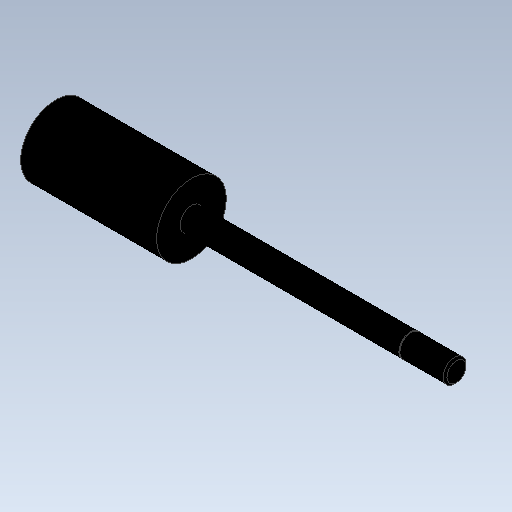
# Autodesk Inventor part: C-041.50000_rod
Saved by Autodesk Inventor 2020 (Build 240168000, 168)
## iProperties
Part Number: C-041.50000_rod
Material: Generic
Catalog Web Link: www.cadenas.de
Description: Standard Air Cylinder_rod-Original Line - Standard Air Cylinders
Vendor: BIMBA
Document SubType Name: Modeling
Designer: partserver
Manufacturer: BIMBA
Mass: 13.1943 g
Surface Area: 43.0398 cm^2
Volume: 13.1943 cm^3
Density: 1 g/cm^3
Appearance: PSOLRGB-0-0-0
Category: PARTsolutions
Company: BIMBA
PSOL_IDENT_0: {$CADENAS_DATA\23d-libs\bimba\bimba_brand\bimba_imperial\bimba_full_line\original_line_cylinders\sta
PSOL_IDENT_1: ndard_air_cylinders\rod.prj},331 {VTYP=3D},{NB=C-041.50000_rod},{LINA=C-041.50000_rod},{NN=Standard
PSOL_IDENT_2: Air Cylinder_rod},{DATE=19.01.2022 10:19:37},{GEOMDATE=27.08.2019 11:00:52},{VERSION=},{LINEID=50},{
PSOL_IDENT_3: WBVAR=STROKE,ACTING,MNT,DER,NR,BM,CO,M,EE,EEL,K,Q,Y,F,G,T,B,H,SER,SR,NT,W,E,HL,ST,STP,PRC,PB,COLOR1,
PSOL_IDENT_4: FCD,RCD,BCD,ZHJ},{WBNUMERIC=STROKE,EEL,COLOR1,FCD,RCD,BCD,ZHJ}  {NB=C-041.50000_rod},{LINA=C-041.500
PSOL_IDENT_5: 00_rod},{KT=DUMMY},{PN=C-041.5000},{DASH=},{BORE=0.75000000},{BOREPN=04},{STROKE=1.500},{STROKEALG=[
PSOL_IDENT_6: 0.001:50/0.001]},{STROKE1=1.500},{ACTING=},{ACTINGALG= '' , 'Single Acting' , 'R' , 'Reverse Single
PSOL_IDENT_7: Acting' , 'D' , 'Double Acting' },{ACTINGPN=},{MNT=},{MNTALG= '' , 'Front Nose Mounting' , 'P' , 'Re
PSOL_IDENT_8: ar Pivot Mounting' , 'BF' , 'Front Block Mounting' , 'BR' , 'Rear Block Mounting for Vertical Positi
PSOL_IDENT_9: oning' , 'BFT' , 'Front Block Trunnion Mounting' , 'BRT' , 'Rear Block Trunnion Mounting' , 'A' , 'D
PSOL_IDENT_10: ouble End Mounting with Brackets and Adjustable Stroke' , 'AP' , 'Rear Pivot Mounting with Adjustabl
PSOL_IDENT_11: e Stroke' },{TYPE=C-},{MNTPN=},{DER=},{DERALG= '' , 'N/A' },{NR=},{NRALG= '' , 'Standard' , 'NR' , '
PSOL_IDENT_12: Non-rotating - Hexagon Rod' },{NRPN=},{BM=},{BMALG= '' , 'Without Built-in Midget 3-Way Solenoid Ope
PSOL_IDENT_13: rated Valve' , 'LS' , 'With Built-in Midget 3-Way Solenoid Operated Valve' },{BMPN=},{CO=},{COALG= ''
PSOL_IDENT_14: , 'N/A' },{M=},{MALG= '', 'Without Magnet', 'M', 'With Magnet' },{EE=},{EEL=0},{EEMAX=10},{EEALG= ''
PSOL_IDENT_15: , 'Without Extra Extension', 'EE', 'With Extra Extension' },{EELALG=0},{EEPN=},{EEPN1=0.000},{K=},{K
PSOL_IDENT_16: ALG= '' , 'N/A' },{KPN=},{Q=},{QALG= '' , 'Without Side Ported Rear Head' , 'Q' , 'With Side Ported
PSOL_IDENT_17: Rear Head' },{QPN=},{Y=},{YALG= '' , 'N/A' },{YPN=},{F=},{FALG= '', 'Standard', 'F', 'Molycoated Bod
PSOL_IDENT_18: y' },{FPN=},{G=},{GPN=},{T=},{TALG= '' , 'Standard' , 'N' , 'Low Temperature' , 'V' , 'High Temperat
PSOL_IDENT_19: ure' },{NPN=},{VPN=},{B=},{BALG= '', 'Without Bumper' , 'B' , 'With Bumper' },{BPN=},{H=},{HALG= '',
PSOL_IDENT_20: 'Standard', 'H', 'With Heavy Springs' },{HPN=},{SER=},{SERALG= '' , 'N/A' },{SR=C},{SRALG= 'C' , 'C
PSOL_IDENT_21: arbon Steel Rod' , 'SR' , '303 Stainless Steel Rod' , '' , '303 Stainless Steel Rod1' },{SRPN=C},{SR
PSOL_IDENT_22: CON=1},{NT=},{NTPN=},{W=},{WALG= '' , 'N/A' },{WPN=},{E=},{EALG= '' , 'Without Special Lube and Seal
PSOL_IDENT_23: s' , 'E' , 'With Special Lube and Seals' },{EPN=},{HL=},{HLALG= '' , 'N/A' },{ST=},{STALG= '' , 'Wit
PSOL_IDENT_24: hout Switch Track' , 'T' , 'With Switch Track' },{STP=},{STPALG= '' , 'N/A' },{STPN=},{PRC=},{PRCALG=
PSOL_IDENT_25: '' , 'Without Piston Rod Clevis' , 'D-166-1' , 'With Piston Rod Clevis' },{PRCPN=},{PB=},{PBALG= ''
PSOL_IDENT_26: , 'Without Pivot Bracket' , 'D-167' , 'With Pivot Bracket' },{PBPN=},{TLEN=3.4460},{TEXT=0.2},{SPAC
PSOL_IDENT_27: E=0.114286},{FRAC=4.3800},{RGCON=},{RGDACCON=},{RHCON=},{RHCONON=1},{RHACCON=},{FNUTCON=1},{RNUTCON=
PSOL_IDENT_28: 0},{FNUTPN=D-98},{RNUTPN=},{FNUTTRANS=0.0000},{RNUTTRANS=0.0000},{VHOLECON=2},{A1=0.8750},{A1N=0.875
PSOL_IDENT_29: 0},{A1P=1.5940},{A1B=1.5940},{A4=0.3130},{A4N=0.3130},{A4P=0.2525},{A5=0.0300},{A1H=0.531},{A1NH=0.5
PSOL_IDENT_30: 310},{A1PH=1.5940},{A1BH=1.0940},{A1SH=1.2190},{A2H=0.2190},{A2NH=0.2190},{LENGTH=1.5000},{LENGTH1=1
PSOL_IDENT_31: .5000},{LENGTH2=3.0300},{MUL=2.5350},{MUL11=2.5350},{MUL22=4.0350},{MUL33=2.5350},{MUL2=1.6900},{MUL
PSOL_IDENT_32: 211=1.6900},{MUL222=2.6900},{MUL233=1.6900},{SSS=3.0000},{RGLEN=0.5920},{RHLEN=0.3420},{SSS1=2.0000}
PSOL_IDENT_33: ,{A13=1.3120},{THDLEN1=0.5000},{THD1=0.2500},{TAB=UNF},{THDLEN=0.5000},{THD=0.2500},{OD=0.7615},{ROD
PSOL_IDENT_34: L=4.3490},{PL=1.4740},{RODDIA=0.2500},{HEX=0.2500},{RODTRANS=0.0000},{G1=0.1250},{ON=0},{G5=0.6250},
PSOL_IDENT_35: {DERLEN=2.8750},{THOLE=0.0000},{WF=0.2200},{BADD=0.0000},{MADD=0.0000},{NVADD=0.000},{JRADD=0.00000}
PSOL_IDENT_36: ,{COLOR=0.00,0.00,0.00,0.00},{GROOVE=1},{HOL=0},{D7=0.2520},{H1=1.1175},{D1=0.8050},{D1RH=0.8050},{D
PSOL_IDENT_37: 1P=0.8325},{D1B=0.8625},{D1N=0.8050},{D1NRH=0.8050},{D1BRH=0.8325},{D1PRH=0.8625},{BOZO=0},{HADD=0.0
PSOL_IDENT_38: 00},{COLOR1=0},{DEFL=0.0000},{HEXL=0.0000},{SSADD=0.0000},{WFL=0.0000},{MOVE=0.0000},{PRCL2=0.50000}
PSOL_IDENT_39: ,{PRCB=0.16000},{PRCTRANS=0.16000},{FCD=0},{RCD=0},{BCD=0},{ZHJ=0.000}
NB: C-041.50000_rod
NN: Standard Air Cylinder_rod
NT: Standard
NBSYN: $PN.$COLOR1._rod
LINA: C-041.50000_rod
CATALOG: Bimba Products
PN: C-041.5000
BORE: 0.75
BOREPN: 04
STROKE: 1.5
ACTING: Single Acting
MNT: Front Nose Mounting
DER: N/A
NR: Standard
BM: Without Built-in Midget 3-Way Solenoid Operated Valve
CO: N/A
M: Without Magnet
EE: Without Extra Extension
EEL: 0
K: N/A
Q: Without Side Ported Rear Head
Y: N/A
F: Standard
G: Without Magnalube Lubrication
T: Standard
B: Without Bumper
H: Standard
SER: N/A
SR: Carbon Steel Rod
W: N/A
E: Without Special Lube and Seals
HL: N/A
ST: Without Switch Track
STP: N/A
PRC: Without Piston Rod Clevis
PB: Without Pivot Bracket
A1N: 0.875
A1P: 1.594
A1B: 1.594
A4N: 0.313
A4P: 0.2525
A5: 0.03
A1NH: 0.531
A1PH: 1.594
A1BH: 1.094
A1SH: 1.219
A2NH: 0.219
A13: 1.312
THDLEN1: 0.5
THD1: 0.25
TAB: UNF
OD: 0.7615
RODDIA: 0.25
HEX: 0.25
G1: 0.125
G5: 0.625
THOLE: 0
WF: 0.22
GROOVE: 1
D7: 0.252
D1P: 0.8325
D1B: 0.8625
D1N: 0.805
D1NRH: 0.805
D1BRH: 0.8325
D1PRH: 0.8625
COLOR1: 0
FCD: 0
RCD: 0
BCD: 0
ZHJ: 0
SUPPLIER: BIMBA
ARTICLENO: C-041.50000_rod
BOMINFO: C-041.50000_rod
CREATOR: CADENAS GmbH
Title: C-041.50000_rod
Author: Cadenas PARTsolutions
Comments: Original Line - Standard Air Cylinders
Autodesk Inventor part; units mm, degrees
ref_plane "YZ Plane" through (0, 0, 0) normal (1, 0, 0) x (0, 1, 0)
ref_plane "XZ Plane" through (0, 0, 0) normal (0, 1, 0) x (-1, 0, 0)
ref_plane "XY Plane" through (0, 0, 0) normal (0, 0, 1) x (1, 0, 0)
sketch "Sketch_1" plane through (0, 0, 0) normal (0, 0, 1) x (1, 0, 0)
  line L0 (97.7646, 0) -> (0, 0)
  line L1 (0, 0) -> (0, 3.175)
  line L2 (0, 3.175) -> (60.325, 3.175)
  line L3 (60.325, 3.175) -> (60.325, 9.6202)
  line L4 (60.325, 9.6202) -> (97.7646, 9.6202)
  line L5 (97.7646, 9.6202) -> (97.7646, 0)
  line L6 (97.7646, 0) -> (0, 0)
  constraints: 14 end point
revolve "Revolution1" add sketch "Sketch_1" angle 360 about axis through (97.7646, 0, 0) along (1, 0, 0)
sketch "Sketch_3" plane through (0, 0, 0) normal (0, 0, 1) x (1, 0, 0)
  line L0 (0, 0) -> (-12.7, 0)
  line L1 (-12.7, 0) -> (-12.7, 2.634)
  line L2 (-12.7, 2.634) -> (-12.159, 3.175)
  line L3 (-12.159, 3.175) -> (0, 3.175)
  line L4 (0, 3.175) -> (0, 0)
  line L5 (0, 0) -> (-12.7, 0)
  constraints: 12 end point
revolve "Revolution2" add sketch "Sketch_3" angle 360 about axis through (0, 0, 0) along (1, 0, 0)
sketch "Sketch_30" plane through (0, 0, 0) normal (0, 0, 1) x (1, 0, 0)
  line L0 (0, 0) -> (-0.254, 0)
  line L1 (-0.254, 2.921) -> (0, 2.921)
  line L2 (0, 2.921) -> (0, 3.429)
  line L3 (0, 3.429) -> (-0.254, 3.429)
  line L4 (-0.254, 3.429) -> (-0.254, 2.921)
  constraints: 10 end point
revolve "Revolution3" cut sketch "Sketch_30" angle 360 about axis through (0, 0, 0) along (1, 0, 0)
ref_plane "dia1_XY" through (0, 3.175, 0) normal (1, 0, 0) x (0, 0, -1)
ref_plane "dia1_YZ" through (0, 3.175, 0) normal (0, 0, -1) x (0, 1, 0)
ref_plane "dia1_ZX" through (0, 3.175, 0) normal (0, 1, 0) x (1, 0, 0)
ref_plane "dia12_XY" through (0, 0, 10.2235) normal (1, 0, 0) x (0, 0, -1)
ref_plane "dia12_YZ" through (0, 0, 10.2235) normal (0, 0, -1) x (0, 1, 0)
ref_plane "dia12_ZX" through (0, 0, 10.2235) normal (0, 1, 0) x (1, 0, 0)
ref_plane "dia2_XY" through (0, -3.175, 0) normal (1, 0, 0) x (0, 0, -1)
ref_plane "dia2_YZ" through (0, -3.175, 0) normal (0, 0, -1) x (0, 1, 0)
ref_plane "dia2_ZX" through (0, -3.175, 0) normal (0, 1, 0) x (1, 0, 0)
ref_plane "dia22_XY" through (0, 0, -10.2235) normal (1, 0, 0) x (0, 0, -1)
ref_plane "dia22_YZ" through (0, 0, -10.2235) normal (0, 0, -1) x (0, 1, 0)
ref_plane "dia22_ZX" through (0, 0, -10.2235) normal (0, 1, 0) x (1, 0, 0)
ref_plane "rl1_XY" through (-12.7, 0, 0) normal (1, 0, 0) x (0, 0, -1)
ref_plane "rl1_YZ" through (-12.7, 0, 0) normal (0, 0, -1) x (0, 1, 0)
ref_plane "rl1_ZX" through (-12.7, 0, 0) normal (0, 1, 0) x (1, 0, 0)
ref_plane "rl2_XY" through (0, 0, 0) normal (1, 0, 0) x (0, 0, -1)
ref_plane "rl2_YZ" through (0, 0, 0) normal (0, 0, -1) x (0, 1, 0)
ref_plane "rl2_ZX" through (0, 0, 0) normal (0, 1, 0) x (1, 0, 0)
ref_plane "rod_cp_XY" through (0, 0, 0) normal (1, 0, 0) x (0, 0, -1)
ref_plane "rod_cp_YZ" through (0, 0, 0) normal (0, 0, -1) x (0, 1, 0)
ref_plane "rod_cp_ZX" through (0, 0, 0) normal (0, 1, 0) x (1, 0, 0)
ref_plane "thd1_XY" through (-12.7, 3.175, 0) normal (1, 0, 0) x (0, 0, -1)
ref_plane "thd1_YZ" through (-12.7, 3.175, 0) normal (0, 0, -1) x (0, 1, 0)
ref_plane "thd1_ZX" through (-12.7, 3.175, 0) normal (0, 1, 0) x (1, 0, 0)
ref_plane "thd2_XY" through (-12.7, -3.175, 0) normal (1, 0, 0) x (0, 0, -1)
ref_plane "thd2_YZ" through (-12.7, -3.175, 0) normal (0, 0, -1) x (0, 1, 0)
ref_plane "thd2_ZX" through (-12.7, -3.175, 0) normal (0, 1, 0) x (1, 0, 0)
ref_plane "to_rod_clevis_XY" through (-16.764, 0, 0) normal (1, 0, 0) x (0, 0, -1)
ref_plane "to_rod_clevis_YZ" through (-16.764, 0, 0) normal (0, 0, -1) x (0, 1, 0)
ref_plane "to_rod_clevis_ZX" through (-16.764, 0, 0) normal (0, 1, 0) x (1, 0, 0)
body "Solid1"
